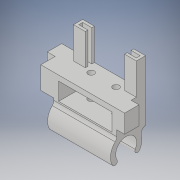
# Autodesk Inventor part: Roller_Switch _30_new
Saved by Autodesk Inventor 2019 (Build 230136000, 136)
## iProperties
Created: 2019-10-10
Part Number: Roller_Switch _30_new
Material: Generic
Document SubType Name: Modeling
Designer: James
Density: 1 g/cm^3
Appearance: Default
Author: James
Autodesk Inventor part; units mm, degrees
ref_plane "YZ Plane" through (0, 0, 0) normal (1, 0, 0) x (0, 1, 0)
ref_plane "XZ Plane" through (0, 0, 0) normal (0, 1, 0) x (-1, 0, 0)
ref_plane "XY Plane" through (0, 0, 0) normal (0, 0, 1) x (1, 0, 0)
sketch "Sketch1" plane through (0, 0, 0) normal (1, 0, 0) x (0, 1, 0)
  circle A0 centre (0, 0) radius 4
  arc A1 (-3, -5.1962) -> (-3, 5.1962) centre (0, 0) ccw
  arc A2 (-3, 5.1962) -> (-2, 3.4641) centre (-2.5, 4.3301) ccw
  arc A3 (-2, -3.4641) -> (-3, -5.1962) centre (-2.5, -4.3301) ccw
  line L0 (15, 3.6) -> (4, 3.6)
  line L1 (4, 3.6) -> (4, -7.4)
  line L2 (4, -7.4) -> (15, -7.4)
  line L3 (15, -7.4) -> (15, 3.6)
  dimension "d0" = 8
  dimension "d1" = 12
  dimension "d2" = 2.5
  dimension "d4" = 11
  dimension "d5" = 11
  dimension "d6" = 4
  dimension "d9" = 7.4
  constraints: 8 end point, 8 point on circle, 4 centre point, 4 tangent, 2 coincident, 2 parallel, 1 horizontal, 1 perpendicular, 1 vertical alignment
  measures "d0" diameter of A0
  measures "d1" diameter of A1
  measures "d2" horizontal distance of A3.centre point (0, 0)
  measures "d4" distance of L2.end L0.start
  measures "d5" distance of L0.start L0.end
  measures "d6" distance from line of point (0, 0) L1
  measures "d9" distance from line of point (0, 0) L2
extrude "Extrusion1" add sketch "Sketch1" along normal blind 24 contours L1 A1 A3 A0 | A0 A2 A1 L0 L1 | L1 L0 A1 | A1 L0 L3 L2 L1
sketch "Sketch2" plane through (0, 4.8, 3.6) normal (0, 0, 1) x (1, 0, 0)
  line L0 (1.8, 8.2) -> (22.2, 8.2)
  line L1 (22.2, 8.2) -> (22.2, 1.5)
  line L2 (22.2, 1.5) -> (1.8, 1.5)
  line L3 (1.8, 1.5) -> (1.8, 8.2)
  line L4 (0, 10.2) -> (24, 10.2) projected
  point P0 (0, -4.8)
  point P1 (12, 8.2)
  point P2 (12, 10.2)
  dimension "d10" = 20.4
  dimension "d11" = 6.7
  dimension "d12" = 13
  constraints: 8 end point, 2 midpoint, 2 parallel, 1 horizontal, 1 perpendicular, 1 vertical alignment
  measures "d10" distance of L0.start L0.end
  measures "d11" distance of L2.end L0.start
  measures "d12" distance from line of point (0, -4.8) L0
extrude "Extrusion2" cut sketch "Sketch2" against normal blind 10
fillet "Fillet1" radius 2 1 edges at (12, 4, -4.4721)
fillet "Fillet2" radius 2 1 edges at (12, 4.8, 3.6)
sketch "Sketch3" plane through (0, 4.8, -6.4) normal (0, 0, 1) x (1, 0, 0)
  line L0 (1.8, 8.2) -> (22.2, 8.2) projected
  line L1 (22.2, 0.9418) -> (1.8, 0.9418) projected
  line L2 (2.2, 8.2) -> (5.4, 8.2)
  line L3 (5.4, 8.2) -> (5.4, 0.9418)
  line L4 (5.4, 0.9418) -> (2.2, 0.9418)
  line L5 (2.2, 0.9418) -> (2.2, 8.2)
  line L6 (11, 8.2) -> (14.2, 8.2)
  line L7 (14.2, 8.2) -> (14.2, 0.9418)
  line L8 (14.2, 0.9418) -> (11, 0.9418)
  line L9 (11, 0.9418) -> (11, 8.2)
  line L10 (18.3, 8.2) -> (21.5, 8.2)
  line L11 (21.5, 8.2) -> (21.5, 0.9418)
  line L12 (21.5, 0.9418) -> (18.3, 0.9418)
  line L13 (18.3, 0.9418) -> (18.3, 8.2)
  line L14 (1.8, 1.5) -> (1.8, 8.2) projected
  point P0 (0, -4.8)
  point P1 (3.8, 8.2)
  point P2 (12.6, 8.2)
  point P3 (19.9, 8.2)
  point P4 (1.8, 1.1156)
  dimension "d17" = 3.2
  dimension "d18" = 3.2
  dimension "d19" = 3.2
  dimension "d20" = 2
  dimension "d21" = 8.8
  dimension "d22" = 7.3
  constraints: 24 end point, 6 parallel, 6 point on line, 3 horizontal, 3 midpoint, 3 perpendicular
  measures "d17" distance between parallel lines of L3 L5
  measures "d18" distance between parallel lines of L7 L9
  measures "d19" distance between parallel lines of L11 L13
  measures "d20" distance from line of point (3.8, 8.2) L14
  measures "d21" distance of point (12.6, 8.2) point (3.8, 8.2)
  measures "d22" distance of point (19.9, 8.2) point (12.6, 8.2)
extrude "Extrusion3" cut sketch "Sketch3" against normal blind 10 contours L0 L3 L1 L5 | L0 L7 L1 L9 | L0 L11 L1 L13
sketch "Sketch4" plane through (0, 15, 3.6) normal (0, 1, 0) x (1, 0, 0)
  circle A0 centre (7.25, 7) radius 1.2
  circle A1 centre (16.75, 7) radius 1.2
  line L0 (0, 11) -> (24, 11) projected
  point P0 (0, 3.6)
  point P1 (12, 11)
  dimension "d25" = 2.4
  dimension "d26" = 9.5
  dimension "d27" = 4.75
  dimension "d28" = 4
  constraints: 2 centre point, 1 equal radius, 1 horizontal alignment, 1 midpoint
  measures "d25" diameter of A0
  measures "d26" distance of A1.centre A0.centre
  measures "d27" horizontal distance of point (12, 11) A0.centre
  measures "d28" distance from line of A0.centre L0
extrude "Extrusion4" cut sketch "Sketch4" against normal blind 10.5
sketch "Sketch5" plane through (24, 0, 0) normal (1, 0, 0) x (0, 0, -1)
  line L0 (-3.6, 15) -> (-3.6, 5.7131) projected
  line L1 (-3.6, 15) -> (1.9, 15)
  line L2 (1.9, 15) -> (1.9, 8)
  line L3 (1.9, 8) -> (-3.6, 8)
  line L4 (-3.6, 8) -> (-3.6, 15)
  point P0 (0, 0)
  dimension "d31" = 5.5
  dimension "d32" = 7
  constraints: 8 end point, 2 parallel, 1 horizontal, 1 perpendicular
  measures "d31" distance of L0.start L1.end
  measures "d32" distance of L1.end L2.end
extrude "Extrusion5" add sketch "Sketch5" along normal blind 3
sketch "Sketch11" plane through (0, 0, 0) normal (-1, 0, 0) x (0, 0, 1)
  line L0 (-7.4, 15) -> (3.6, 15) projected
  line L1 (3.6, 15) -> (3.6, 5.7131) projected
  line L2 (-7.4, 15) -> (3.6, 15)
  line L3 (3.6, 15) -> (3.6, 6.5)
  line L4 (3.6, 6.5) -> (-7.4, 6.5)
  line L5 (-7.4, 6.5) -> (-7.4, 15)
  point P0 (0, 0)
  constraints: 8 end point, 2 parallel, 2 point on line, 1 horizontal, 1 perpendicular
extrude "Extrusion10" add sketch "Sketch11" along normal blind 5
sketch "Sketch12" plane through (-5, 0, 0) normal (-1, 0, 0) x (0, 0, 1)
  line L0 (-7.4, 15) -> (-7.4, 6.5) projected
  line L1 (-1.9, 15) -> (-1.9, 8) projected
  line L2 (-7.4, 15) -> (-1.9, 15)
  line L3 (-1.9, 15) -> (-1.9, 8)
  line L4 (-1.9, 8) -> (-7.4, 8)
  line L5 (-7.4, 8) -> (-7.4, 15)
  point P0 (0, 0)
  dimension "d63" = 5.5
  dimension "d64" = 7
  constraints: 8 end point, 2 parallel, 1 horizontal, 1 perpendicular
  measures "d63" distance of L1.end L4.end
  measures "d64" distance of L2.end L1.end
extrude "Extrusion11" add sketch "Sketch12" along normal blind 3
sketch "Sketch13" plane through (24, 15, -1.9) normal (0, 1, 0) x (1, 0, 0)
  line L0 (-24, 5.5) -> (0, 5.5) projected
  line L1 (-4.5, 5.5) -> (0, 5.5)
  line L2 (0, 5.5) -> (0, 0) projected
  line L3 (-4.5, 2) -> (-4.5, 3)
  line L4 (-4.5, 3) -> (-1, 3)
  line L5 (-1, 3) -> (-1, 4.5)
  line L6 (-1, 4.5) -> (-4.5, 4.5)
  line L7 (-4.5, 4.5) -> (-4.5, 5.5)
  line L8 (-24, -5.5) -> (-24, 5.5) projected
  line L9 (-24, 2) -> (-19.5, 2)
  line L10 (-19.5, 2) -> (-19.5, 3)
  line L11 (-19.5, 3) -> (-23, 3)
  line L12 (-23, 3) -> (-23, 4.5)
  line L13 (-23, 4.5) -> (-19.5, 4.5)
  line L14 (-19.5, 4.5) -> (-19.5, 5.5)
  line L15 (-18.6, 5.5) -> (-21.8, 5.5) projected
  line L16 (-19.5, 5.5) -> (-24, 5.5)
  line L17 (-4.5, 2) -> (0, 2)
  line L18 (0, 3.8385) -> (0, 5.5) projected
  line L19 (0, 2) -> (0, 5.5)
  line L20 (-24, 3.8385) -> (-24, 5.5) projected
  line L21 (-24, 2) -> (-24, 5.5)
  point P0 (-24, -1.9)
  point P1 (0, 3.9038)
  point P2 (-24, 3.9038)
  point P3 (-2.25, 2)
  point P4 (-21.75, 2)
  dimension "d67" = 3.5
  dimension "d68" = 1.5
  dimension "d69" = 1
  dimension "d70" = 1
  dimension "d71" = 4.5
  dimension "d72" = 4.5
  constraints: 32 end point, 11 point on line, 7 perpendicular, 3 collinear, 3 vertical, 2 midpoint, 1 horizontal, 1 horizontal alignment
  measures "d67" distance between parallel lines of L1 L17
  measures "d68" distance of L4.end L5.end
  measures "d69" distance between parallel lines of L2 L5
  measures "d70" distance between parallel lines of L8 L12
  measures "d71" distance of L3.start L17.end
  measures "d72" distance of L9.start L9.end
extrude "Extrusion12" add sketch "Sketch13" along normal blind 12
body "Solid1"
